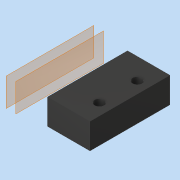
# Autodesk Inventor part: Limit Switch
Saved by Autodesk Inventor 2017 SP1 (Build 210196100, 196)
## iProperties
Created: 2018-12-30
Part Number: Limit Switch
Material: ABS Plastic
Document SubType Name: Modeling
Designer: Dylan Rice
Density: 1.06 g/cm^3
Appearance: Smooth - White(1)
Author: Dylan Rice
Autodesk Inventor part; units mm, degrees
ref_plane "YZ Plane" through (0, 0, 0) normal (1, 0, 0) x (0, 1, 0)
ref_plane "XZ Plane" through (0, 0, 0) normal (0, 1, 0) x (-1, 0, 0)
ref_plane "XY Plane" through (0, 0, 0) normal (0, 0, 1) x (1, 0, 0)
sketch "Sketch1" plane through (0, 0, 0) normal (0, 1, 0) x (-1, 0, 0)
  line L0 (0, 41.1799) -> (0, -51.3986) construction
  line L1 (10.6, 10) -> (0, 10)
  line L2 (0, 10) -> (0, -10)
  line L3 (0, -10) -> (10.6, -10)
  line L4 (10.6, -10) -> (10.6, 10)
  circle A0 centre (2.9, 4.75) radius 1.2
  line L5 (10.6, 0) -> (0, 0) construction
  circle A1 centre (2.9, -4.75) radius 1.2
  dimension "d0" = 10.6
  dimension "d1" = 20
  dimension "d2" = 2.9
  dimension "d3" = 2.4
  dimension "d4" = 9.5
  constraints: 12 end point, 2 centre point, 2 midpoint, 2 parallel, 1 horizontal, 1 perpendicular, 1 point on line, 1 symmetric about line, 1 vertical, 1 other
  measures "d0" distance between parallel lines of L4 L2
  measures "d1" distance between parallel lines of L3 L1
  measures "d2" distance from line of L0 A0.centre
  measures "d3" diameter of A0
  measures "d4" distance of A1.centre A0.centre
extrude "Extrusion1" add sketch "Sketch1" along normal blind 6.4
ref_plane "Rolling Contact Plane" through (-20, 0, 10) normal (1, 0, 0) x (0, 0, -1)
ref_plane "Trigger Plane" through (-17.6, 0, 10) normal (1, 0, 0) x (0, 0, -1)
body "Solid1"
